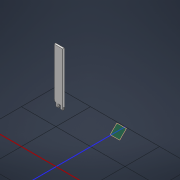
# Autodesk Inventor part: frame-roof
Saved by Autodesk Inventor 2021 (Build 250183000, 183)
## iProperties
Created: 2020-05-07
Part Number: frame-roof
Material: Generic
Document SubType Name: Modeling
Designer: Jonathan
Density: 1 g/cm^3
Appearance: Default
Author: Jonathan
Autodesk Inventor part; units mm, degrees
ref_plane "YZ Plane" through (0, 0, 0) normal (1, 0, 0) x (0, 1, 0)
ref_plane "XZ Plane" through (0, 0, 0) normal (0, 1, 0) x (-1, 0, 0)
ref_plane "XY Plane" through (0, 0, 0) normal (0, 0, 1) x (1, 0, 0)
sketch "Sketch1" plane through (0, 0, 0) normal (0, 1, 0) x (-1, 0, 0)
  line L0 (0, 0.5) -> (-25, 0.5)
  line L1 (-25, 0.5) -> (-25, 5.5)
  line L2 (-25, 5.5) -> (0, 5.5)
  line L3 (0, 5.5) -> (0, 0.5)
  line L4 (-5, 0) -> (0, 0) projected
  line L5 (-25, 0) -> (-5, 0) projected
  dimension "d0" = 5
  dimension "d1" = 0.5
  constraints: 8 end point, 2 perpendicular, 2 vertical alignment, 1 horizontal, 1 parallel
  measures "d0" distance of L2.end L0.start
  measures "d1" distance between parallel lines of L0 L5
extrude "Extrusion1" add sketch "Sketch1" along normal blind 150
ref_plane "Work Plane1" through (12.5, -150.2602, -167.9379) normal (0, -0.7071068, -0.7071068) x (-1, 0, 0)
sketch "Sketch2" plane through (12.5, -150.2602, -167.9379) normal (0, -0.7071068, -0.7071068) x (-1, 0, 0)
  arc A0 (7.5, -12.5) -> (12.5, -7.5) centre (7.5, -7.5) ccw projected
  line L0 (12.5, 12.5) -> (12.5, -7.5) projected
  line L1 (7.5, -12.5) -> (-12.5, -12.5) projected
  line L2 (12.5, 12.5) -> (27.4723, 12.5)
  line L3 (27.4723, 12.5) -> (27.4723, -26.1223)
  line L4 (27.4723, -26.1223) -> (-16.9009, -26.1223)
  line L5 (-16.9009, -26.1223) -> (-16.9009, -12.5)
  line L6 (-16.9009, -12.5) -> (-12.5, -12.5)
  point P0 (12.5, -12.5)
  constraints: 10 end point, 3 perpendicular, 1 horizontal
extrude "Extrusion2" cut sketch "Sketch2" against normal through all
sketch "Sketch3" plane through (0, 150, 5.5) normal (0, 0, 1) x (1, 0, 0)
  line L0 (5, -144.5) -> (25, -144.5) projected
  line L1 (5, -144.5) -> (5, -154.5)
  line L2 (5, -154.5) -> (25, -154.5)
  line L3 (25, -144.5) -> (25, 0) projected
  line L4 (25, -154.5) -> (25, -144.5)
  point P0 (0, -150)
  dimension "d8" = 10
  constraints: 6 end point, 2 perpendicular, 1 vertical
  measures "d8" distance of L0.start L1.end
extrude "Extrusion3" add sketch "Sketch3" against normal blind 3
sketch "Sketch4" plane through (25, 150, 5.5) normal (1, 0, 0) x (0, 0, -1)
  line L0 (0, -144.5) -> (0, -154.5) projected
  line L1 (5, -149.5) -> (5, -142.4289) projected
  line L2 (3, -147.5) -> (5, -149.5) projected
  line L3 (3.1066, -152) -> (5.3033, -149.8033) construction
  line L4 (164.599, -309.099) -> (5.5, -150) projected
  circle A0 centre (3.1066, -152) radius 2.5
  line L5 (3.1066, -152) -> (0, -152) construction
  line L6 (3.1066, -152) -> (3.1066, -154.5) construction
  point P0 (3, -154.5)
  dimension "d9" = 5
  constraints: 6 end point, 2 perpendicular, 2 point on line, 1 coincident, 1 equal length, 1 horizontal alignment, 1 vertical, 1 vertical alignment, 2 other
extrude "Extrusion4" add sketch "Sketch4" against normal up to surface (20 mm away)
sketch "Sketch5" plane through (25, 150, 5.5) normal (1, 0, 0) x (0, 0, -1)
  arc A0 (3, -154.4977) -> (3, -149.5023) centre (3.1066, -152) ccw projected
  circle A1 centre (3.1066, -152) radius 1.5
  point P0 (5.5, -150)
  dimension "d12" = 1
  constraints: 1 centre point, 1 coincident
  measures "d12" radial gap between concentric circles of A0 A1
extrude "Extrusion5" cut sketch "Sketch5" against normal through all
sketch "Sketch6" plane through (5, -4.5, 5.5) normal (0, -1, 0) x (1, 0, 0)
  line L0 (6.6667, -5.6066) -> (13.3333, -5.6066)
  line L1 (13.3333, -5.6066) -> (13.3333, -1.6066)
  line L2 (13.3333, -1.6066) -> (6.6667, -1.6066)
  line L3 (6.6667, -1.6066) -> (6.6667, -5.6066)
  line L4 (0, -5.6066) -> (0, -3) projected
  line L5 (20, -3) -> (0, -3) construction
  line L6 (0, -3) -> (20, -3) construction
  line L7 (10, -5.6066) -> (10, -1.6066) construction
  line L8 (20, -1.6066) -> (20, -4.6066) construction
  line L9 (20, -5.6066) -> (20, -3) construction
  point P0 (-5, -5.5)
  point P1 (10, -3)
  dimension "d15" = 6.6667
  constraints: 12 end point, 4 midpoint, 2 horizontal, 2 horizontal alignment, 2 parallel, 2 perpendicular, 2 point on line
  measures "d15" distance of L0.start L0.end
extrude "Extrusion6" cut sketch "Sketch6" against normal blind 4
sketch "Sketch9" plane through (12.5, -150.2602, -167.9379) normal (0, -0.7071068, -0.7071068) x (-1, 0, 0)
  line L0 (0.8333, -12.5) -> (-5.8333, -12.5)
  line L1 (-5.8333, -12.5) -> (-5.8333, -19.5711)
  line L2 (-5.8333, -19.5711) -> (0.8333, -19.5711)
  line L3 (0.8333, -19.5711) -> (0.8333, -12.5)
  line L4 (0.8333, -17.4497) -> (0.8333, -18.435) projected
  line L5 (-5.8333, -18.435) -> (-5.8333, -17.4497) projected
  point P0 (12.5, -12.5)
  point P1 (0.8333, -17.9424)
  point P2 (-5.8333, -17.9424)
  point P3 (7.5, -19.5711)
  point P4 (-12.5, -12.5)
  constraints: 8 end point, 4 point on line, 2 midpoint, 2 parallel, 1 horizontal, 1 perpendicular
extrude "Extrusion7" cut sketch "Sketch9" against normal through all
fillet "Fillet1" radius 0.5 6 edges at (21.6667, -4.5, 5.5) (8.3333, -4.5, 5.5) (11.6667, 0.5, 5.5) (18.3333, 0.5, 5.5) (5, 0.5, 5.5) (15, 5.5, 5.5)
fillet "Fillet1" radius 1 3 edges at (0, 81.2855, 5.5) (1.4645, 7.5711, 5.5) (25, 72.75, 5.5)
equation "\"d16\" = d9 - d12"
body "Solid1"
